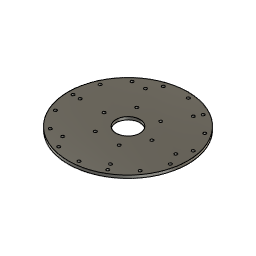
MID_LAYER_v2 (Autodesk Fusion 360 design; units mm, degrees)
Autodesk Fusion 360 part; units mm, degrees
sketch "Sketch1" plane through (0, 0, 0) normal (0, 0, 1) x (1, 0, 0)
  circle A0 centre (0, 0) radius 125
  line L0 (0, 0) -> (125, 0)
  line L1 (0, 0) -> (-62.5, 108.2532)
  line L2 (0, 0) -> (-62.5, -108.2532)
  line L3 (0, 0) -> (125, 0) construction
  line L4 (0, 0) -> (100, 0)
  line L5 (0, 0) -> (50, 0)
  line L6 (0, 0) -> (-3.1039, 5.3762)
  line L7 (0, 0) -> (-25, 43.3013)
  line L8 (-25, 43.3013) -> (-50, 86.6025)
  line L9 (0, 0) -> (-25, -43.3013)
  line L10 (-25, -43.3013) -> (-50, -86.6025)
  line L11 (0, 0) -> (62.5, -108.2532)
  line L12 (0, 0) -> (125, 0) construction
  line L13 (0, 0) -> (-125, 0)
  line L14 (0, 0) -> (62.5, 108.2532)
  circle A1 centre (-25, 43.3013) radius 3
  circle A2 centre (-50, 86.6025) radius 3
  circle A3 centre (50, 0) radius 3
  circle A4 centre (100, 0) radius 3
  circle A5 centre (-25, -43.3013) radius 3
  circle A6 centre (-50, -86.6025) radius 3
  line L15 (0, 0) -> (-100, 0)
  line L16 (0, 0) -> (2.1092, 3.6532)
  line L17 (0, 0) -> (50, 86.6025)
  line L18 (0, 0) -> (50, -86.6025)
  circle A7 centre (50, -86.6025) radius 3
  circle A8 centre (25, -43.3013) radius 3
  circle A9 centre (-50, 0) radius 3
  circle A10 centre (-100, 0) radius 3
  line L19 (0, 0) -> (50, 86.6025)
  circle A11 centre (25, 43.3013) radius 3
  circle A12 centre (50, 86.6025) radius 3
  line L20 (-125, 0) -> (-115, 0)
  circle A13 centre (-115, 0) radius 3
  circle A14 centre (-105.0577, -46.7747) radius 3
  circle A15 centre (-76.95, -85.4617) radius 3
  circle A16 centre (-35.537, -109.3715) radius 3
  circle A17 centre (12.0208, -114.37) radius 3
  circle A18 centre (57.5, -99.5929) radius 3
  circle A19 centre (93.037, -67.5953) radius 3
  circle A20 centre (112.487, -23.9098) radius 3
  circle A21 centre (112.487, 23.9098) radius 3
  circle A22 centre (93.037, 67.5953) radius 3
  circle A23 centre (57.5, 99.5929) radius 3
  circle A24 centre (12.0208, 114.37) radius 3
  circle A25 centre (-35.537, 109.3715) radius 3
  circle A26 centre (-76.95, 85.4617) radius 3
  circle A27 centre (-105.0577, 46.7747) radius 3
  dimension "d1" = 250
  dimension "d2" = 60
  dimension "d3" = 120
  dimension "d4" = 100
  dimension "d5" = 50
  dimension "d6" = 50
  dimension "d7" = 50
  dimension "d8" = 50
  dimension "d9" = 50
  dimension "d10" = 60
  dimension "d11" = 60
  dimension "d12" = 6
  dimension "d13" = 6
  dimension "d14" = 6
  dimension "d15" = 6
  dimension "d16" = 6
  dimension "d17" = 6
  dimension "d18" = 100
  dimension "d19" = 100
  dimension "d20" = 100
  dimension "d21" = 6
  dimension "d22" = 6
  dimension "d23" = 6
  dimension "d24" = 6
  dimension "d25" = 100
  dimension "d26" = 6
  dimension "d27" = 6
  dimension "d28" = 10
  dimension "d29" = 6
  dimension "d31" = 360
  constraint coincident A0.centre L0.start
  constraint coincident A0 L0.end
  constraint horizontal L0
  constraint horizontal L3
  constraint parallel L0 L4
  constraint parallel L3 L5
  constraint coincident L1 L6.end
  constraint parallel L1 L6
  constraint parallel L1 L7
  constraint parallel L1 L8
  constraint parallel L2 L9
  constraint parallel L2 L10
  constraint horizontal L12
  constraint coincident A0 L13.end
  constraint horizontal L13
  constraint coincident L7.end L8.start
  constraint coincident L8.end A2.centre
  constraint coincident L5.end A3.centre
  constraint coincident L4.end A4.centre
  constraint coincident L9.end L10.start
  constraint coincident L10.end A6.centre
  constraint parallel L13 L15
  constraint coincident L14 L16.end
  constraint parallel L14 L17
  constraint parallel L11 L18
  constraint coincident L18.end A7.centre
  constraint midpoint L18 A8.centre
  constraint midpoint L15 A9.centre
  constraint coincident L15.end A10.centre
  constraint parallel L17 L19
  constraint midpoint L19 A11.centre
  constraint coincident L17.end L19.end
  constraint parallel L13 L20
  constraint coincident L20.end A13.centre
  measures "d1" diameter of A0
  measures "d2" angle of L0 L1
  measures "d3" angle of L2 L3
  measures "d4" distance of A0.centre L4.end
  measures "d5" distance of A0.centre L5.end
  measures "d6" distance of A0.centre L7.end
  measures "d7" distance of L7.end L8.end
  measures "d8" distance of A0.centre L9.end
  measures "d9" distance of L9.end L10.end
  measures "d10" angle of L11 L12
  measures "d11" angle of L13 L14
  measures "d12" diameter of A1
  measures "d13" diameter of A2
  measures "d14" diameter of A3
  measures "d15" diameter of A4
  measures "d16" diameter of A5
  measures "d17" diameter of A6
  measures "d18" distance of A0.centre L15.end
  measures "d19" distance of A0.centre L17.end
  measures "d20" distance of A0.centre L18.end
  measures "d21" diameter of A7 L6.end
  measures "d22" diameter of A8 L6.end
  measures "d23" diameter of A9
  measures "d24" diameter of A10
  measures "d25" distance of A0.centre L17.end
  measures "d26" diameter of A11 L6.end
  measures "d27" diameter of A12 L6.end
  measures "d28" distance of L13.end L20.end
  measures "d29" diameter of A13
extrude "Extrude1" add sketch "Sketch1" along normal blind 6 contours A0 L0 L4 L5 L14 A3 A4 L16 L17 L19 A11 A12 A23 | A0 L0 L4 L5 L11 A3 A4 L18 A7 A8 A18 | A0 L1 L6 L7 L8 L14 A1 A2 L16 L17 L19 A11 A12 A23 | A0 L2 L9 L10 L11 A5 A6 L18 A7 A8 A18 | A0 L1 L6 L7 L8 L13 A1 A2 L15 A9 A10 L20 A13 | A0 L2 L9 L10 L13 A5 A6 L15 A9 A10 L20 A13
sketch "Sketch2" plane through (0, 0, 6) normal (0, 0, 1) x (-1, 0, 0)
  circle A0 centre (-93.037, 67.5953) radius 3
  circle A1 centre (-25, -43.3013) radius 3
  circle A2 centre (105.0577, -46.7747) radius 3
  circle A3 centre (50, 0) radius 3
  circle A4 centre (-50, -86.6025) radius 3
  circle A5 centre (105.0577, 46.7747) radius 3
  circle A6 centre (25, 43.3013) radius 3
  circle A7 centre (-57.5, 99.5929) radius 3
  circle A8 centre (-93.037, -67.5953) radius 3
  circle A9 centre (76.95, 85.4617) radius 3
  circle A10 centre (-57.5, -99.5929) radius 3
  circle A11 centre (50, 86.6025) radius 3
  circle A12 centre (-112.487, 23.9098) radius 3
  circle A13 centre (35.537, -109.3715) radius 3
  circle A14 centre (-12.0208, -114.37) radius 3
  circle A15 centre (-112.487, -23.9098) radius 3
  circle A16 centre (50, -86.6025) radius 3
  circle A17 centre (76.95, -85.4617) radius 3
  circle A18 centre (-50, 0) radius 3
  circle A19 centre (-100, 0) radius 3
  circle A20 centre (100, 0) radius 3
  circle A21 centre (115, 0) radius 3
  circle A22 centre (-50, 86.6025) radius 3
  circle A23 centre (-12.0208, 114.37) radius 3
  circle A24 centre (35.537, 109.3715) radius 3
  circle A25 centre (25, -43.3013) radius 3
  circle A26 centre (-25, 43.3013) radius 3
  circle A27 centre (0, 0) radius 125
  circle A28 centre (0, 0) radius 25
  constraint coincident A27.centre A28.centre
extrude "Extrude2" cut sketch "Sketch2" against normal blind 6 contours A28
